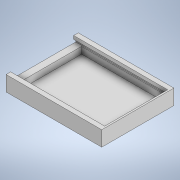
# Autodesk Inventor part: TapaCajaArduinoNano
Saved by Autodesk Inventor 2021 (Build 250183000, 183)
## iProperties
Created: 2020-09-06
Part Number: TapaCajaArduinoNano
Material: Genérico
Document SubType Name: Modeling
Designer: igtw1
Density: 1 g/cm^3
Appearance: Valor por defecto
Author: igtw1
Autodesk Inventor part; units mm, degrees
ref_plane "YZ Plane" through (0, 0, 0) normal (1, 0, 0) x (0, 1, 0)
ref_plane "XZ Plane" through (0, 0, 0) normal (0, 1, 0) x (-1, 0, 0)
ref_plane "XY Plane" through (0, 0, 0) normal (0, 0, 1) x (1, 0, 0)
sketch "Boceto1" plane through (0, 0, 0) normal (0, 1, 0) x (-1, 0, 0)
  line L0 (28.5, 20.5) -> (-28.5, 20.5)
  line L1 (-28.5, 20.5) -> (-28.5, -20.5)
  line L2 (-28.5, -20.5) -> (28.5, -20.5)
  line L3 (28.5, -20.5) -> (28.5, 20.5)
  line L4 (28.5, 20.5) -> (-28.5, -20.5) construction
  line L5 (-28.5, 20.5) -> (28.5, -20.5) construction
  point P0 (0, 0)
  dimension "d0" = 57
  dimension "d1" = 41
  constraints: 12 end point, 2 midpoint, 2 parallel, 1 horizontal, 1 perpendicular
  measures "d0" distance of L2.end L1.end
  measures "d1" distance of L1.end L0.end
extrude "Extrusión1" add sketch "Boceto1" along normal blind 8
sketch "Boceto2" plane through (0, 8, 0) normal (0, 1, 0) x (1, 0, 0)
  line L0 (28.5, -20.5) -> (28.5, 20.5) projected
  line L1 (28.5, -20.5) -> (28.5, -17.5)
  line L2 (28.5, -17.5) -> (26.5, -17.5)
  line L3 (26.5, -17.5) -> (26.5, 17.5)
  line L4 (28.5, 20.5) -> (-28.5, 20.5) projected
  line L5 (26.5, 17.5) -> (-24.5, 17.5)
  line L6 (-24.5, 17.5) -> (-24.5, -17.5)
  line L7 (-24.5, -17.5) -> (26.5, -17.5)
  point P0 (0, 0)
  dimension "d4" = 3
  dimension "d5" = 2
  dimension "d6" = 35
  dimension "d7" = 51
  constraints: 12 end point, 4 perpendicular, 1 horizontal, 1 point on line
  measures "d4" distance of L0.start L1.end
  measures "d5" distance of L1.end L2.end
  measures "d6" distance of L2.end L3.end
  measures "d7" distance of L3.end L5.end
extrude "Extrusión2" cut sketch "Boceto2" against normal blind 6
sketch "Boceto3" plane through (0, 8, 0) normal (0, 1, 0) x (1, 0, 0)
  line L0 (-24.5, -17.5) -> (-24.5, 17.5) projected
  line L1 (-24.5, -17.5) -> (-28.5, -17.5)
  line L2 (-28.5, 20.5) -> (-28.5, -20.5) projected
  line L3 (-28.5, -17.5) -> (-28.5, 17.5)
  line L4 (-24.5, 17.5) -> (26.5, 17.5) projected
  line L5 (-28.5, 17.5) -> (-24.5, 17.5)
  line L6 (-24.5, 17.5) -> (-24.5, -17.5)
  point P0 (0, 0)
  dimension "d10" = 35
  constraints: 8 end point, 1 horizontal, 1 perpendicular, 1 point on line
  measures "d10" distance of L1.end L3.end
extrude "Extrusión3" cut sketch "Boceto3" against normal blind 6
sketch "Boceto4" plane through (-28.5, 0, -20.5) normal (-1, 0, 0) x (0, 0, 1)
  line L0 (3, 8) -> (38, 8) projected
  line L1 (3, 8) -> (3, 7)
  line L2 (3, 7) -> (2, 7)
  line L3 (2, 7) -> (2, 6)
  line L4 (2, 6) -> (3, 6)
  line L5 (3, 8) -> (3, 2) projected
  line L6 (3, 6) -> (3, 7)
  point P0 (20.5, 0)
  dimension "d13" = 1
  dimension "d14" = 1
  dimension "d15" = 1
  constraints: 10 end point, 3 perpendicular, 1 horizontal, 1 point on line, 1 vertical
  measures "d13" distance of L0.start L1.end
  measures "d14" distance of L1.end L2.end
  measures "d15" distance of L2.end L3.end
extrude "Extrusión4" cut sketch "Boceto4" against normal blind 55
sketch "Boceto5" plane through (-28.5, 0, -20.5) normal (-1, 0, 0) x (0, 0, 1)
  line L0 (3, 8) -> (38, 8) projected
  line L1 (38, 8) -> (38, 7)
  line L2 (38, 8) -> (38, 2) projected
  line L3 (38, 7) -> (39, 7)
  line L4 (39, 7) -> (39, 6)
  line L5 (39, 6) -> (38, 6)
  line L6 (38, 7) -> (38, 6)
  point P0 (20.5, 0)
  dimension "d18" = 1
  dimension "d19" = 1
  dimension "d20" = 1
  constraints: 10 end point, 4 perpendicular, 2 point on line
  measures "d18" distance of L0.end L1.end
  measures "d19" distance of L1.end L3.end
  measures "d20" distance of L3.end L4.end
extrude "Extrusión5" cut sketch "Boceto5" against normal blind 55
sketch "Boceto6" plane through (-28.5, 0, -20.5) normal (-1, 0, 0) x (0, 0, 1)
  line L0 (3, 8) -> (3, 7) projected
  line L1 (3, 8) -> (3, 6)
  line L2 (3, 6) -> (1, 6)
  line L3 (1, 6) -> (1, 7)
  line L4 (2, 6) -> (2, 7) projected
  line L5 (1, 7) -> (2, 7)
  line L6 (2, 7) -> (2, 8)
  line L7 (0, 8) -> (3, 8) projected
  line L8 (3, 8) -> (2, 8)
  point P0 (20.5, 0)
  dimension "d23" = 2
  dimension "d24" = 2
  dimension "d25" = 1
  constraints: 12 end point, 3 perpendicular, 1 collinear, 1 point on line
  measures "d23" distance of L0.start L1.end
  measures "d24" distance of L1.end L2.end
  measures "d25" distance of L2.end L3.end
extrude "Extrusión6" cut sketch "Boceto6" against normal blind 55
sketch "Boceto7" plane through (-28.5, 0, -20.5) normal (-1, 0, 0) x (0, 0, 1)
  line L0 (2, 8) -> (38, 8) projected
  line L1 (39, 6) -> (38, 6) projected
  line L2 (38, 8) -> (38, 6)
  line L3 (38, 6) -> (40, 6)
  line L4 (40, 6) -> (40, 7)
  line L5 (38, 7) -> (39, 7) projected
  line L6 (40, 7) -> (39, 7)
  line L7 (39, 7) -> (39, 8)
  line L8 (38, 8) -> (41, 8) projected
  line L9 (38, 8) -> (39, 8)
  point P0 (20.5, 0)
  dimension "d28" = 2
  dimension "d29" = 1
  constraints: 12 end point, 4 perpendicular, 1 collinear, 1 point on line
  measures "d28" distance of L1.end L3.end
  measures "d29" distance of L3.end L4.end
extrude "Extrusión7" cut sketch "Boceto7" against normal blind 55
sketch "Boceto8" plane through (26.5, 2, -17.5) normal (-1, 0, 0) x (0, 0, 1)
  line L0 (-1, 6) -> (36, 6) projected
  line L1 (-1, 5) -> (-1, 6) projected
  line L2 (-1, 6) -> (-1, 5)
  line L3 (-2, 4) -> (-2, 5) projected
  line L4 (-1, 5) -> (-2, 5)
  line L5 (-2, 5) -> (-2, 4)
  line L6 (0, 4) -> (-2, 4) projected
  line L7 (-2, 4) -> (0, 4)
  line L8 (0, 0) -> (0, 4) projected
  line L9 (0, 4) -> (0, 0)
  line L10 (35, 4) -> (35, 0) projected
  line L11 (0, 0) -> (35, 0)
  line L12 (35, 0) -> (35, 4)
  line L13 (37, 4) -> (35, 4) projected
  line L14 (35, 4) -> (37, 4)
  line L15 (37, 5) -> (37, 4) projected
  line L16 (37, 4) -> (37, 5)
  line L17 (36, 5) -> (37, 5) projected
  line L18 (37, 5) -> (36, 5)
  line L19 (36, 6) -> (36, 5) projected
  line L20 (36, 5) -> (36, 6)
  line L21 (36, 6) -> (-1, 6)
  point P0 (17.5, -2)
  constraints: 24 end point, 8 perpendicular, 3 collinear, 1 vertical
extrude "Extrusión8" cut sketch "Boceto8" against normal blind 1
sketch "Boceto9" plane through (-28.5, 0, -20.5) normal (-1, 0, 0) x (0, 0, 1)
  line L0 (3, 2) -> (3, 6) projected
  line L1 (3, 6) -> (3, 2)
  line L2 (38, 2) -> (3, 2) projected
  line L3 (3, 2) -> (38, 2)
  line L4 (38, 6) -> (38, 2) projected
  line L5 (38, 2) -> (38, 6)
  line L6 (38, 6) -> (3, 6)
  point P0 (20.5, 0)
  constraints: 8 end point, 2 collinear, 1 perpendicular, 1 vertical
extrude "Extrusión9" add sketch "Boceto9" against normal blind 4
sketch "Boceto10" plane through (-28.5, 0, -20.5) normal (-1, 0, 0) x (0, 0, 1)
  line L0 (0, 0) -> (41, 0) projected
  line L1 (0, 0) -> (42, 0)
  line L2 (42, 0) -> (42, 8)
  line L3 (42, 8) -> (42, 9)
  line L4 (42, 9) -> (40, 9)
  line L5 (40, 9) -> (40, 7)
  line L6 (40, 7) -> (41, 7)
  line L7 (41, 0) -> (41, 8) projected
  line L8 (41, 7) -> (41, 5)
  line L9 (41, 5) -> (0, 5)
  line L10 (0, 0) -> (0, 8) projected
  line L11 (0, 5) -> (0, 7)
  line L12 (1, 7) -> (2, 7) projected
  line L13 (0, 7) -> (1, 7)
  line L14 (1, 7) -> (1, 9)
  line L15 (1, 9) -> (-1, 9)
  line L16 (-1, 9) -> (-1, 0)
  line L17 (-1, 0) -> (0, 0)
  point P0 (20.5, 0)
  dimension "d36" = 42
  dimension "d37" = 8
  dimension "d38" = 1
  dimension "d39" = 2
  dimension "d40" = 2
  dimension "d41" = 2
  constraints: 28 end point, 10 perpendicular, 4 point on line, 1 collinear, 1 vertical
  measures "d36" distance of L0.start L1.end
  measures "d37" distance of L1.end L2.end
  measures "d38" distance of L2.end L3.end
  measures "d39" distance of L4.end L5.end
  measures "d40" distance of L6.end L8.end
  measures "d41" distance of L14.end L15.end
extrude "Extrusión10" add sketch "Boceto10" against normal blind 57
sketch "Boceto11" plane through (-28.5, 6, -19.5) normal (-1, 0, 0) x (0, 0, 1)
  line L0 (39, 2) -> (0, 2) projected
  line L1 (39, 2) -> (39, 1)
  line L2 (38, 1) -> (39, 1) projected
  line L3 (39, 1) -> (38, 1)
  line L4 (38, 2) -> (38, 1) projected
  line L5 (38, 1) -> (38, 2)
  line L6 (38, 2) -> (39, 2)
  line L7 (0, 1) -> (1, 1) projected
  line L8 (0, 1) -> (0, 2)
  line L9 (1, 1) -> (1, 2) projected
  line L10 (0, 2) -> (1, 2)
  line L11 (1, 2) -> (1, 1)
  line L12 (0, 0) -> (0, 1) projected
  line L13 (1, 1) -> (0, 1)
  line L14 (0, 1) -> (-1, 1)
  line L15 (-1, 1) -> (-1, -1)
  line L16 (-1, -1) -> (40, -1)
  line L17 (41, 3) -> (41, -6) projected
  line L18 (40, -1) -> (40, 1)
  line L19 (40, 1) -> (39, 1)
  line L20 (0, 1) -> (1, 1) projected
  line L21 (0, 0) -> (0, 1) projected
  line L22 (0, 1) -> (0, 0)
  line L23 (0, 0) -> (39, 0)
  line L24 (39, 0) -> (39, 1)
  line L25 (39, 1) -> (39, 0) projected
  line L26 (39, 1) -> (39, 0)
  point P0 (19.5, -6)
  dimension "d44" = 1
  dimension "d45" = 2
  dimension "d46" = 41
  constraints: 34 end point, 13 perpendicular, 2 point on line, 2 vertical, 1 collinear
  measures "d44" distance of L7.start L14.end
  measures "d45" distance of L14.end L15.end
  measures "d46" distance of L15.end L16.end
extrude "Extrusión11" cut sketch "Boceto11" against normal blind 56 contours L1 L2 L4 L0 | L19 L18 L16 L15 L14 L12 L23 L24 | L9 L7 L8 L0
sketch "Boceto12" plane through (28.5, 0, 21.5) normal (1, 0, 0) x (0, 0, -1)
  line L0 (2, 8) -> (2, 9) projected
  line L1 (41, 9) -> (41, 8) projected
  line L2 (2, 8) -> (41, 8)
  line L3 (41, 8) -> (41, 9)
  line L4 (41, 9) -> (2, 9)
  line L5 (2, 9) -> (2, 8)
  point P0 (21.5, 0)
  constraints: 8 end point, 2 parallel, 1 horizontal, 1 perpendicular
extrude "Extrusión12" add sketch "Boceto12" against normal blind 1
sketch "Boceto13" plane through (-28.5, 5, 20.5) normal (0, 1, 0) x (1, 0, 0)
  line L0 (56, 1) -> (56, 0) projected
  line L1 (0, 40) -> (56, 40) projected
  line L2 (56, 1) -> (4, 1)
  line L3 (4, 1) -> (4, 40)
  line L4 (4, 40) -> (56, 40)
  line L5 (56, 40) -> (56, 1)
  point P0 (28.5, 20.5)
  dimension "d51" = 52
  constraints: 8 end point, 2 parallel, 1 horizontal, 1 perpendicular, 1 point on line
  measures "d51" distance of L3.end L4.end
extrude "Extrusión13" cut sketch "Boceto13" against normal blind 4
sketch "Boceto14" plane through (-28.5, 0, -21.5) normal (-1, 0, 0) x (0, 0, 1)
  line L0 (41, 9) -> (2, 9) projected
  line L1 (41, 9) -> (40.25, 9)
  line L2 (40.25, 9) -> (40.25, 7)
  line L3 (40.25, 7) -> (41.5, 7)
  line L4 (41, 7) -> (42, 7) projected
  line L5 (41.5, 7) -> (41.5, 5)
  line L6 (41, 5) -> (42, 5) projected
  line L7 (41.5, 5) -> (1.5, 5)
  line L8 (41, 5) -> (2, 5) projected
  line L9 (1.5, 5) -> (1.5, 7)
  line L10 (1, 7) -> (2, 7) projected
  line L11 (1.5, 7) -> (2.75, 7)
  line L12 (2.75, 7) -> (2.75, 9)
  line L13 (0, 9) -> (43, 9) projected
  line L14 (2.75, 9) -> (0, 9)
  line L15 (0, 0) -> (0, 9) projected
  line L16 (0, 9) -> (0, 0)
  line L17 (43, 9) -> (43, 0) projected
  line L18 (0, 0) -> (43, 0)
  line L19 (43, 0) -> (43, 9)
  line L20 (43, 9) -> (40.25, 9)
  point P0 (21.5, 0)
  point P1 (2, 7)
  dimension "d54" = 0.75
  dimension "d55" = 2
  dimension "d56" = 40
  dimension "d57" = 1.25
  constraints: 26 end point, 4 perpendicular, 4 point on line, 3 collinear, 3 midpoint, 1 vertical
  measures "d54" distance of L0.start L1.end
  measures "d55" distance of L1.end L2.end
  measures "d56" distance of L5.end L7.end
  measures "d57" distance of L9.end L11.end
extrude "Extrusión14" add sketch "Boceto14" against normal blind 4 contours L13 L17 L18 L15 L0 L12 L11 L10 L9 L7 L6 L5 L3 L2
sketch "Boceto15" plane through (-24.5, 0, -21.5) normal (1, 0, 0) x (0, 0, -1)
  line L0 (-2.75, 9) -> (-2.75, 7) projected
  line L1 (-2.75, 9) -> (-2, 9)
  line L2 (-2, 9) -> (-2, 7)
  line L3 (-2.75, 7) -> (-2, 7) projected
  line L4 (-2, 7) -> (-2.75, 7)
  line L5 (-2.75, 7) -> (-2.75, 9)
  line L6 (-1, 5) -> (-1.5, 5) projected
  line L7 (-1.5, 5) -> (-1, 5)
  line L8 (-1, 7) -> (-1, 5) projected
  line L9 (-1, 5) -> (-1, 7)
  line L10 (-1, 7) -> (-1.5, 7)
  line L11 (-1.5, 7) -> (-1.5, 5) projected
  line L12 (-1.5, 7) -> (-1.5, 5)
  line L13 (-41, 7) -> (-41, 9) projected
  line L14 (-40.25, 9) -> (-41, 9) projected
  line L15 (-41, 9) -> (-40.25, 9)
  line L16 (-40.25, 7) -> (-40.25, 9) projected
  line L17 (-40.25, 9) -> (-40.25, 7)
  line L18 (-41, 7) -> (-40.25, 7) projected
  line L19 (-40.25, 7) -> (-41, 7)
  line L20 (-41, 7) -> (-41, 9)
  line L21 (-41.5, 5) -> (-42, 5) projected
  line L22 (-41.5483, 5) -> (-42, 5)
  line L23 (-42, 5) -> (-42, 7) projected
  line L24 (-42, 5) -> (-42, 7)
  line L25 (-42, 7) -> (-41.5, 7) projected
  line L26 (-42, 7) -> (-41.5, 7)
  line L27 (-41.5, 5) -> (-41.5, 7) projected
  line L28 (-41.5, 7) -> (-41.5, 5)
  point P0 (-21.5, 0)
  constraints: 32 end point, 6 collinear, 6 perpendicular, 3 horizontal
extrude "Extrusión15" add sketch "Boceto15" along normal blind 53
